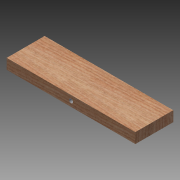
# Autodesk Inventor part: CNC-1.1v-X-4-(plate form mover)
Saved by Autodesk Inventor 2015 (Build 190159000, 159)
## iProperties
Created: 2015-07-10
Part Number: CNC-1.1v-X-4-(plate form mover)
Material: Generic
Document SubType Name: Modeling
Designer: Bangladesh
Density: 1 g/cm^3
Appearance: Default
Author: Bangladesh
Autodesk Inventor part; units mm, degrees
ref_plane "YZ Plane" through (0, 0, 0) normal (1, 0, 0) x (0, 1, 0)
ref_plane "XZ Plane" through (0, 0, 0) normal (0, 1, 0) x (-1, 0, 0)
ref_plane "XY Plane" through (0, 0, 0) normal (0, 0, 1) x (1, 0, 0)
sketch "Sketch1" plane through (0, 0, 0) normal (1, 0, 0) x (0, 1, 0)
  line L0 (19.05, 69.85) -> (-19.05, 69.85)
  line L1 (-19.05, 69.85) -> (-19.05, -69.85)
  line L2 (-19.05, -69.85) -> (19.05, -69.85)
  line L3 (19.05, -69.85) -> (19.05, 69.85)
  line L4 (19.05, 69.85) -> (-19.05, -69.85) construction
  line L5 (-19.05, 69.85) -> (19.05, -69.85) construction
  point P0 (0, 0)
  dimension "d0" = 38.1
  dimension "d1" = 139.7
  constraints: 12 end point, 2 midpoint, 2 parallel, 1 horizontal, 1 perpendicular
  measures "d0" distance of L2.end L1.end
  measures "d1" distance of L1.end L0.end
extrude "Extrusion1" add sketch "Sketch1" along normal mid plane 474
sketch "Sketch2" plane through (-237, -19.05, 69.85) normal (0, 0, 1) x (1, 0, 0)
  circle A0 centre (237, 19.05) radius 7.165
  dimension "d4" = 14.33
  constraints: 1 centre point, 1 coincident
  measures "d4" diameter of A0
hole "Hole1" at (0, 0, 69.85) direction (0, 0, -1) diameter 14.3 end through all
body "Solid1"
